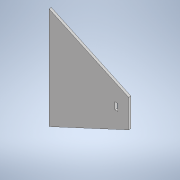
# Autodesk Inventor part: Pata
Saved by Autodesk Inventor 2020.1 (Build 241239000, 239)
## iProperties
Created: 2019-12-03
Part Number: Pata
Material: Generic
Document SubType Name: Modeling
Designer: Daniel
Density: 1 g/cm^3
Appearance: Default
Author: Daniel
Autodesk Inventor part; units mm, degrees
ref_plane "YZ Plane" through (0, 0, 0) normal (1, 0, 0) x (0, 1, 0)
ref_plane "XZ Plane" through (0, 0, 0) normal (0, 1, 0) x (-1, 0, 0)
ref_plane "XY Plane" through (0, 0, 0) normal (0, 0, 1) x (1, 0, 0)
sketch "Sketch1" plane through (0, 0, 0) normal (0, 0, 1) x (1, 0, 0)
  line L0 (0, -54) -> (0, 0) construction
  line L1 (0.7624, -54) -> (19.2963, -45.3931) projected
  line L2 (-85, 39.8266) -> (-85, -93.8266)
  line L3 (1.7624, -31) -> (1.7624, -23) projected
  line L4 (5.2624, -31.5) -> (1.2624, -31.5)
  line L5 (1.2624, -31.5) -> (1.2624, -22.5)
  line L6 (1.2624, -22.5) -> (5.2624, -22.5)
  line L7 (5.2624, -22.5) -> (5.2624, -31.5)
  line L8 (19.2963, -45.3931) -> (19.2963, -8.6069) projected
  line L9 (0.7624, 0) -> (19.2963, -8.6069) projected
  line L10 (19.2963, -8.6069) -> (-85, 39.8266)
  line L11 (19.2963, -45.3931) -> (-85, -93.8266)
  line L12 (19.2963, -8.6069) -> (19.2963, -45.3931)
  line L13 (4.7624, -23) -> (4.7624, -31) projected
  line L14 (4.7624, -31) -> (1.7624, -31) projected
  line L15 (1.7624, -23) -> (4.7624, -23) projected
  point P0 (0, 0)
  dimension "d0" = 85
  dimension "d5" = 0.5
  dimension "d6" = 0.5
  dimension "d7" = 0.5
  dimension "d8" = 0.5
  constraints: 18 end point, 2 collinear, 2 vertical, 1 other
  measures "d0" distance of the line from the sketch origin of L2
  measures "d5" distance between parallel lines of L4 L14
  measures "d6" distance between parallel lines of L7 L13
  measures "d7" distance between parallel lines of L6 L15
  measures "d8" distance between parallel lines of L3 L5
extrude "Extrusion1" add sketch "Sketch1" along normal blind 3 contours L11 L2 L10 L9 L8 L1
body "Solid1"
